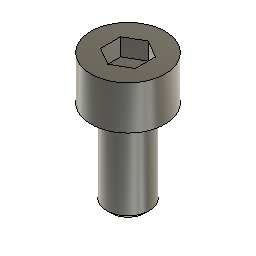
2022-09-05_xz-605-bearing-z-axis-trial (Autodesk Fusion 360 archive; units mm, degrees)
design "HW_M5x10-SHCS"
Autodesk Fusion 360 part; units mm, degrees
sketch "Sketch1" plane through (0, 0, 0) normal (0, 1, 0) x (1, 0, 0)
  line L0 (0, -5) -> (0, 10)
  line L1 (0, 10) -> (1.95, 10)
  line L2 (1.95, 10) -> (2.45, 9.5)
  line L3 (2.45, 9.5) -> (2.45, 0)
  line L4 (2.45, 0) -> (4.25, 0)
  line L5 (4.25, 0) -> (4.25, -5)
  line L6 (4.25, -5) -> (0, -5)
  dimension "d1" = 10
  dimension "d2" = 45
  dimension "d3" = 0.5
  dimension "d4" = 2.45
  dimension "d5" = 5
  dimension "d6" = 4.25
  constraint vertical L0
  constraint perpendicular L0 L1
  constraint perpendicular L1 L3
  constraint perpendicular L3 L4
  constraint perpendicular L4 L5
  constraint horizontal L6
  constraint coincident origin L0
  constraint coincident origin L4
  measures "d1" distance of origin L1
  measures "d2" angle of L1 L2
  measures "d3" horizontal distance of L1.end L2.end
  measures "d4" distance of L0.end L3
  measures "d5" distance of L4.end L5.end
  measures "d6" distance of L0.start L5.end
revolve "Revolve1" add sketch "Sketch1" angle 360 about axis through (0, 0, 5) along (0, 0, -1)
sketch "Sketch2" plane through (0, 0, 5) normal (0, 0, 1) x (-1, 0, 0)
  circle A0 centre (0, 0) radius 4.25
  line L0 (-2, -1.1547) -> (0, -2.3094)
  line L1 (0, -2.3094) -> (2, -1.1547)
  line L2 (2, -1.1547) -> (2, 1.1547)
  line L3 (2, 1.1547) -> (0, 2.3094)
  line L4 (0, 2.3094) -> (-2, 1.1547)
  line L5 (-2, 1.1547) -> (-2, -1.1547)
  dimension "d8" = 4
  constraint coincident A0.centre origin
  constraint vertical L5
  measures "d8" distance of L1.end L5
extrude "Extrude1" cut sketch "Sketch2" against normal blind 2 contours L0 L1 L2 L3 L4 L5
equation "d4 = ( 4.9 / 2 ) * 1 mm"
equation "d6 = ( 8.5 / 2 ) * 1 mm"

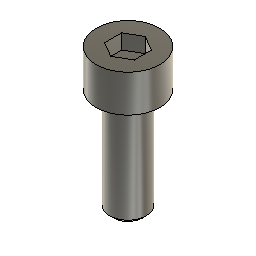
design "HW_M5x14-SHCS"
Autodesk Fusion 360 part; units mm, degrees
sketch "Sketch1" plane through (0, 0, 0) normal (0, 1, 0) x (1, 0, 0)
  line L0 (0, -5) -> (0, 14)
  line L1 (0, 14) -> (1.95, 14)
  line L2 (1.95, 14) -> (2.45, 13.5)
  line L3 (2.45, 13.5) -> (2.45, 0)
  line L4 (2.45, 0) -> (4.25, 0)
  line L5 (4.25, 0) -> (4.25, -5)
  line L6 (4.25, -5) -> (0, -5)
  dimension "d1" = 14
  dimension "d2" = 45
  dimension "d3" = 0.5
  dimension "d4" = 2.45
  dimension "d5" = 5
  dimension "d6" = 4.25
  constraint vertical L0
  constraint perpendicular L0 L1
  constraint perpendicular L1 L3
  constraint perpendicular L3 L4
  constraint perpendicular L4 L5
  constraint horizontal L6
  constraint coincident origin L0
  constraint coincident origin L4
  measures "d1" distance of origin L1
  measures "d2" angle of L1 L2
  measures "d3" horizontal distance of L1.end L2.end
  measures "d4" distance of L0.end L3
  measures "d5" distance of L4.end L5.end
  measures "d6" distance of L0.start L5.end
revolve "Revolve1" add sketch "Sketch1" angle 360 about axis through (0, 0, 5) along (0, 0, -1)
sketch "Sketch2" plane through (0, 0, 5) normal (0, 0, 1) x (-1, 0, 0)
  circle A0 centre (0, 0) radius 4.25
  line L0 (-2, -1.1547) -> (0, -2.3094)
  line L1 (0, -2.3094) -> (2, -1.1547)
  line L2 (2, -1.1547) -> (2, 1.1547)
  line L3 (2, 1.1547) -> (0, 2.3094)
  line L4 (0, 2.3094) -> (-2, 1.1547)
  line L5 (-2, 1.1547) -> (-2, -1.1547)
  dimension "d8" = 4
  constraint coincident A0.centre origin
  constraint vertical L5
  measures "d8" distance of L1.end L5
extrude "Extrude1" cut sketch "Sketch2" against normal blind 2 contours L0 L1 L2 L3 L4 L5
equation "d4 = ( 4.9 / 2 ) * 1 mm"
equation "d6 = ( 8.5 / 2 ) * 1 mm"

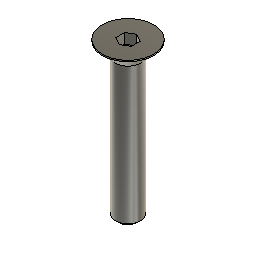
design "HW_M5x30-FHCS"
Autodesk Fusion 360 part; units mm, degrees
sketch "Sketch1" plane through (0, 0, 0) normal (0, 1, 0) x (1, 0, 0)
  line L0 (0, 0) -> (0, 30)
  line L1 (0, 30) -> (1.95, 30)
  line L2 (1.95, 30) -> (2.45, 29.5)
  line L3 (2.45, 29.5) -> (2.45, 2.8)
  line L4 (2.45, 2.8) -> (5, 0.25)
  line L5 (5, 0.25) -> (5, 0)
  line L6 (5, 0) -> (0, 0)
  dimension "d1" = 2.45
  dimension "d3" = 45
  dimension "d5" = 0.5
  dimension "d6" = 30
  dimension "d7" = 5
  dimension "d9" = 0.25
  constraint coincident L0.start L6.end
  constraint vertical L0
  constraint perpendicular L0 L1
  constraint perpendicular L1 L3
  constraint parallel L2 L4
  constraint parallel L3 L5
  constraint perpendicular L5 L6
  measures "d1" distance of L0.end L3
  measures "d3" angle of L1 L2
  measures "d5" distance of L1.end L3
  measures "d6" distance of L0.start L0.end
  measures "d7" distance of L5.end L0.start
  measures "d9" distance of L4.end L5.end
revolve "Revolve1" add sketch "Sketch1" angle 360 about axis through (0, 0, 1.75) along (0, 0, 1)
sketch "Sketch2" plane through (0, 0, 0) normal (0, 0, 1) x (-1, 0, 0)
  circle A0 centre (0, 0) radius 5
  line L0 (-1.5, -0.866) -> (0, -1.7321)
  line L1 (0, -1.7321) -> (1.5, -0.866)
  line L2 (1.5, -0.866) -> (1.5, 0.866)
  line L3 (1.5, 0.866) -> (0, 1.7321)
  line L4 (0, 1.7321) -> (-1.5, 0.866)
  line L5 (-1.5, 0.866) -> (-1.5, -0.866)
  dimension "d12" = 3
  constraint coincident A0.centre origin
  constraint vertical L5
  measures "d12" distance of L2 L5
extrude "Extrude1" cut sketch "Sketch2" against normal blind 2 contours L0 L1 L2 L3 L4 L5
equation "d1 = ( 4.9 / 2 ) * 1 mm"
equation "d7 = ( 10 / 2 ) * 1 mm"

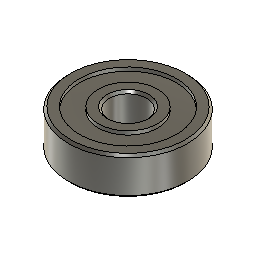
design "PP_BRNG_625-5x16x5"
Autodesk Fusion 360 part; units mm, degrees
sketch "Sketch1" plane through (0, 0, 0) normal (0, 1, 0) x (1, 0, 0)
  line L0 (2.5, -2.5) -> (4, -2.5)
  line L1 (4, 2.5) -> (2.5, 2.5)
  line L2 (2.5, 2.5) -> (2.5, -2.5)
  line L3 (6.5, -2.5) -> (8, -2.5)
  line L4 (8, -2.5) -> (8, 2.5)
  line L5 (8, 2.5) -> (6.5, 2.5)
  line L6 (4, -2) -> (6.5, -2)
  line L7 (4, 2) -> (6.5, 2)
  line L8 (4, -2.5) -> (4, -2)
  line L9 (4, 2) -> (4, 2.5)
  line L10 (6.5, 2.5) -> (6.5, 2)
  line L11 (6.5, -2) -> (6.5, -2.5)
  line L12 (8, 0) -> (0, 0) construction
  point P0 (2.5, 0)
  dimension "d1" = 2.5
  dimension "d2" = 8
  dimension "d4" = 0.5
  dimension "d5" = 5
  dimension "d8" = 1.5
  constraint horizontal L0
  constraint vertical L8
  constraint horizontal L1
  constraint vertical L2
  constraint horizontal L3
  constraint vertical L4
  constraint horizontal L5
  constraint vertical L10
  constraint coincident L6.end L10
  constraint perpendicular L6 L10
  constraint coincident L7.start L8
  constraint perpendicular L7 L8
  constraint collinear L8 L9
  constraint collinear L10 L11
  constraint midpoint L4 L12.start
  constraint coincident L12.end origin
  constraint horizontal L12
  constraint midpoint L2 P0
  constraint coincident L12 P0
  constraint equal L0 L3
  constraint equal L8 L9
  constraint coincident L0 L3.start
  measures "d1" distance of L12.end L2
  measures "d2" distance of L12.end L4
  measures "d4" distance of L0.end L6.start
  measures "d5" distance of L3.end L4.end
  measures "d8" distance of L0.start L0.end
revolve "Revolve1" add sketch "Sketch1" angle 360 about axis through (0, 0, 1.75) along (0, 0, 1)
chamfer "Chamfer1" distance 0.3 angle 45 4 edges at (-2.3308, -0.904, 2.5) (-7.4586, -2.8929, 2.5) (-7.4586, -2.8929, -2.5) (-2.3308, -0.904, -2.5)
equation "d1 = ( 5 / 2 ) * 1 mm"
equation "d2 = ( 16 / 2 ) * 1 mm"

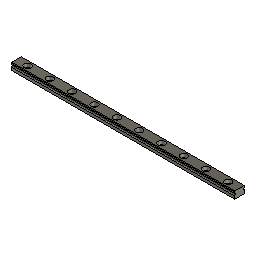
design "PP_BRNG_MGN9-Rail-200"
Autodesk Fusion 360 part; units mm, degrees
sketch "Sketch1" plane through (0, 0, 0) normal (1, 0, 0) x (0, 1, 0)
  line L0 (4.75, 0) -> (-4.75, 0)
  line L1 (-4.75, 0) -> (-4.75, 6.5)
  line L2 (-4.75, 6.5) -> (4.75, 6.5)
  line L3 (4.75, 6.5) -> (4.75, 0)
  circle A0 centre (-4.75, 4) radius 1
  circle A1 centre (4.75, 4) radius 1
  line L4 (4.75, 4) -> (-4.75, 4) construction
  dimension "d1" = 9.5
  dimension "d2" = 6.5
  dimension "d3" = 2
  dimension "d4" = 2.5
  constraint horizontal L0
  constraint vertical L1
  constraint horizontal L2
  constraint vertical L3
  constraint midpoint origin L0
  constraint coincident L1 A0.centre
  constraint coincident L3 A1.centre
  constraint coincident A1.centre L4.start
  constraint coincident A0.centre L4.end
  constraint horizontal L4
  constraint equal A0 A1
  measures "d1" distance of L0.start L0.end
  measures "d2" distance of L0.start L2.end
  measures "d3" diameter of A1
  measures "d4" distance of L1.end L4
extrude "Extrude1" add sketch "Sketch1" along normal blind 200 contours L0 L1 L2 L3 A0 A1
chamfer "Chamfer1" distance 0.5 angle 45 4 edges at (100, 4.75, 6.5) (100, -4.75, 6.5) (100, 4.75, 0) (100, -4.75, 0)
sketch "Sketch2" plane through (0, 0, 0) normal (0, 0, 1) x (1, 0, 0)
  circle A0 centre (10, 0) radius 1.75
  circle A1 centre (10, 0) radius 3
  line L0 (10, 0) -> (0, 0) construction
  dimension "d8" = 3.5
  dimension "d9" = 6
  dimension "d10" = 10
  constraint concentric A0 A1
  constraint coincident A0.centre A1.centre
  constraint coincident L0.end origin
  constraint horizontal L0
  measures "d8" diameter of A0
  measures "d9" diameter of A1
  measures "d10" distance of A0.centre L0.end
extrude "Extrude2" cut sketch "Sketch2" along normal up to surface (6.5 mm away) contours A0
extrude "Extrude3" cut sketch "Sketch2" against normal blind 3.5 from surface at 6.5
pattern_linear "R-Pattern1" count 10 spacing 20 along (1, 0, 0) of "Extrude2", "Extrude3"

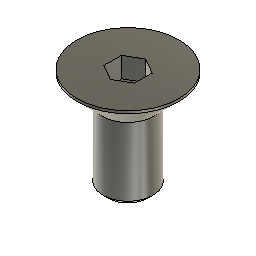
design "HW_M5x10-FHCS"
Autodesk Fusion 360 part; units mm, degrees
sketch "Sketch1" plane through (0, 0, 0) normal (0, 1, 0) x (1, 0, 0)
  line L0 (0, 0) -> (0, 10)
  line L1 (0, 10) -> (1.95, 10)
  line L2 (1.95, 10) -> (2.45, 9.5)
  line L3 (2.45, 9.5) -> (2.45, 2.8)
  line L4 (2.45, 2.8) -> (5, 0.25)
  line L5 (5, 0.25) -> (5, 0)
  line L6 (5, 0) -> (0, 0)
  dimension "d1" = 2.45
  dimension "d3" = 45
  dimension "d5" = 0.5
  dimension "d6" = 10
  dimension "d7" = 5
  dimension "d9" = 0.25
  constraint coincident L0.start L6.end
  constraint vertical L0
  constraint perpendicular L0 L1
  constraint perpendicular L1 L3
  constraint parallel L2 L4
  constraint parallel L3 L5
  constraint perpendicular L5 L6
  measures "d1" distance of L0.end L3
  measures "d3" angle of L1 L2
  measures "d5" distance of L1.end L3
  measures "d6" distance of L0.start L0.end
  measures "d7" distance of L5.end L0.start
  measures "d9" distance of L4.end L5.end
revolve "Revolve1" add sketch "Sketch1" angle 360 about axis through (0, 0, 1.75) along (0, 0, 1)
sketch "Sketch2" plane through (0, 0, 0) normal (0, 0, 1) x (-1, 0, 0)
  circle A0 centre (0, 0) radius 5
  line L0 (-1.5, -0.866) -> (0, -1.7321)
  line L1 (0, -1.7321) -> (1.5, -0.866)
  line L2 (1.5, -0.866) -> (1.5, 0.866)
  line L3 (1.5, 0.866) -> (0, 1.7321)
  line L4 (0, 1.7321) -> (-1.5, 0.866)
  line L5 (-1.5, 0.866) -> (-1.5, -0.866)
  dimension "d12" = 3
  constraint coincident A0.centre origin
  constraint vertical L5
  measures "d12" distance of L2 L5
extrude "Extrude1" cut sketch "Sketch2" against normal blind 2 contours L0 L1 L2 L3 L4 L5
equation "d1 = ( 4.9 / 2 ) * 1 mm"
equation "d7 = ( 10 / 2 ) * 1 mm"
